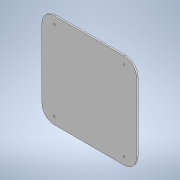
# Autodesk Inventor part: payload_bay_square
Saved by Autodesk Inventor 2020.2 (Build 242310000, 310)
## iProperties
Created: 2020-02-19
Part Number: payload_bay_square
Material: Generic
Document SubType Name: Modeling
Designer: Krishna Makhija
Density: 1 g/cm^3
Appearance: Default
Author: Krishna Makhija
Autodesk Inventor part; units mm, degrees
ref_plane "YZ Plane" through (0, 0, 0) normal (1, 0, 0) x (0, 1, 0)
ref_plane "XZ Plane" through (0, 0, 0) normal (0, 1, 0) x (-1, 0, 0)
ref_plane "XY Plane" through (0, 0, 0) normal (0, 0, 1) x (1, 0, 0)
sketch "Sketch1" plane through (0, 0, 0) normal (0, 0, 1) x (1, 0, 0)
  point P0 (0, 0)
sketch "Sketch2" plane through (0, 0, 0) normal (0, 0, 1) x (1, 0, 0)
  line L0 (94.9998, -95.0001) -> (-94.9998, -95.0001)
  line L1 (-94.9998, -95.0001) -> (-94.9998, 95.0001)
  line L2 (-94.9998, 95.0001) -> (94.9998, 95.0001)
  line L3 (94.9998, 95.0001) -> (94.9998, -95.0001)
  line L4 (94.9998, -95.0001) -> (-94.9998, 95.0001) construction
  line L5 (-94.9998, -95.0001) -> (94.9998, 95.0001) construction
  point P0 (0, 0)
  constraints: 12 end point, 2 midpoint, 2 parallel, 1 horizontal, 1 perpendicular
extrude "Extrusion1" add sketch "Sketch2" along normal blind 3
sketch "Sketch3" plane through (0, 0, 3) normal (0, 0, 1) x (1, 0, 0)
  circle A0 centre (70, 80) radius 1.5001
  circle A1 centre (70, -80) radius 1.5001
  circle A2 centre (-70, 80) radius 1.5001
  circle A3 centre (-70, -80) radius 1.5001
  constraints: 4 centre point
extrude "Extrusion2" cut sketch "Sketch3" against normal blind 3
fillet "Fillet1" radius 25 1 edges at (94.9998, 95.0001, 1.5)
fillet "Fillet2" radius 25 1 edges at (94.9998, -95.0001, 1.5)
fillet "Fillet3" radius 25 1 edges at (-94.9998, -95.0001, 1.5)
fillet "Fillet4" radius 25 1 edges at (-94.9998, 95.0001, 1.5)
body "Solid1"
